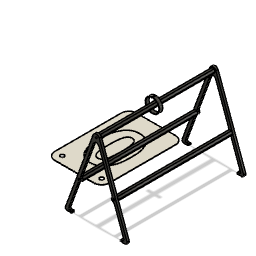
230527 flip scoreboard (Autodesk Fusion 360 design; units mm, degrees)
Autodesk Fusion 360 part; units mm, degrees
sketch "number base" plane through (0, 0, 0) normal (0, 1, 0) x (1, 0, 0)
  line L0 (-14, 0) -> (-86, 0)
  line L1 (-100, -14) -> (-100, -136)
  line L2 (-86, -150) -> (-14, -150)
  line L3 (0, -136) -> (0, -14)
  arc A0 (-14, -150) -> (0, -136) centre (-14, -136) ccw
  arc A1 (-100, -136) -> (-86, -150) centre (-86, -136) ccw
  arc A2 (-86, 0) -> (-100, -14) centre (-86, -14) ccw
  arc A3 (0, -14) -> (-14, 0) centre (-14, -14) ccw
  circle A4 centre (-14, -136) radius 3.5
  circle A5 centre (-86, -136) radius 3.5
  point P0 (-100, 0)
  point P1 (0, -150)
  dimension "d1" = 150
  dimension "d2" = 100
  dimension "d3" = 14
  dimension "d4" = 7
  dimension "d5" = 7
  constraint horizontal L0
  constraint vertical L1
  constraint horizontal L2
  constraint vertical L3
  constraint coincident P1 L2
  constraint coincident P1 L3
  constraint tangent L2 A0
  constraint tangent L3 A0
  constraint tangent L1 A1
  constraint tangent L2 A1
  constraint equal A0 A1
  constraint coincident P0 L0
  constraint coincident P0 L1
  constraint tangent L0 A2
  constraint tangent L1 A2
  constraint equal A0 A2
  constraint coincident origin L0
  constraint coincident origin L3
  constraint tangent L0 A3
  constraint tangent L3 A3
  constraint equal A0 A3
  constraint concentric A0 A4
  constraint concentric A1 A5
  measures "d1" distance of origin P1
  measures "d2" distance of origin P0
  measures "d3" radius of A0
  measures "d4" diameter of A4
  measures "d5" diameter of A5
extrude "Extrude1" add sketch "number base" along normal blind 0.6 makes body 1
sketch "Sketch3" plane through (0, 0.6, 0) normal (0, 1, 0) x (-1, 0, 0)
  circle A0 centre (14, 136) radius 3.5
  circle A1 centre (86, 136) radius 3.5
  arc A2 (0, 14) -> (14, 0) centre (14, 14) ccw
  line L0 (14, 0) -> (86, 0)
  arc A3 (86, 0) -> (100, 14) centre (86, 14) ccw
  line L1 (100, 14) -> (100, 136)
  arc A4 (100, 136) -> (86, 150) centre (86, 136) ccw
  line L2 (86, 150) -> (14, 150)
  arc A5 (14, 150) -> (0, 136) centre (14, 136) ccw
  line L3 (0, 136) -> (0, 14)
  line L4 (0, 75) -> (100, 75)
  line L5 (50, 150) -> (50, 0)
  line L6 (21.099, 26.201) -> (78.901, 26.201) construction
  line L7 (78.901, 26.201) -> (78.901, 123.799) construction
  line L8 (78.901, 123.799) -> (21.099, 123.799) construction
  line L9 (21.099, 123.799) -> (21.099, 26.201) construction
  dimension "d9" = 90
  text T0 "0" font "Arial" height 90 bold align centre middle in box 57.802 x 97.5981 at (21.099, 26.201) x (1, 0) y (0, 1) spacing 1 kerned
  constraint midpoint L3 L4.start
  constraint midpoint L1 L4.end
  constraint midpoint L2 L5.start
  constraint midpoint L0 L5.end
extrude "Extrude2" add sketch "Sketch3" along normal blind 0.4 separate body text T0 makes body 2
combine "Combine1" operation add target body 2 tool bodies 1
sketch "stand" plane through (0, 0, 0) normal (0, 0, 1) x (1, 0, 0)
  line L0 (1.7096, 4.6971) -> (52.5053, 144.257)
  line L1 (4.9985, 0) -> (170, 0) construction
  line L2 (58.1434, 159.7477) -> (58.1434, -80)
  line L3 (4.9985, 0) -> (13, 0)
  line L4 (14, 1) -> (14, 2)
  line L5 (13, 3) -> (9.2691, 3)
  arc A0 (1.7096, 4.6971) -> (4.9985, 0) centre (4.9985, 3.5) ccw
  arc A1 (7.3897, 5.684) -> (9.2691, 3) centre (9.2691, 5) ccw
  arc A2 (14, 2) -> (13, 3) centre (13, 2) ccw
  arc A3 (13, 0) -> (14, 1) centre (13, 1) ccw
  line L6 (103.2868, 3) -> (107.0178, 3)
  arc A4 (103.2868, 3) -> (102.2868, 2) centre (103.2868, 2) ccw
  line L7 (102.2868, 1) -> (102.2868, 2)
  arc A5 (102.2868, 1) -> (103.2868, 0) centre (103.2868, 1) ccw
  line L8 (111.2883, 0) -> (103.2868, 0)
  arc A6 (111.2883, 0) -> (114.5773, 4.6971) centre (111.2883, 3.5) ccw
  line L9 (114.5773, 4.6971) -> (63.7816, 144.257)
  line L10 (108.8971, 5.684) -> (63.3117, 130.9289)
  arc A7 (107.0178, 3) -> (108.8971, 5.684) centre (107.0178, 5) ccw
  arc A8 (63.7816, 144.257) -> (52.5053, 144.257) centre (58.1434, 142.2049) ccw
  arc A9 (63.3117, 130.9289) -> (52.9751, 130.9289) centre (58.1434, 129.0478) ccw
  circle A10 centre (58.1434, 142.2049) radius 1.65
  circle A11 centre (26.0949, 60) radius 1.65
  line L11 (29.1691, 68.4463) -> (23.0207, 51.5537) construction
  line L12 (7.3897, 5.684) -> (24.8987, 53.7896)
  line L13 (29.1705, 65.5264) -> (52.9751, 130.9289)
  arc A12 (27.3762, 56.2108) -> (29.5121, 62.0791) centre (26.0949, 60) ccw
  line L14 (29.8537, 58.6319) -> (32.665, 66.3559) construction
  arc A13 (29.1705, 65.5264) -> (29.5121, 62.0791) centre (32.9293, 64.1583) ccw
  arc A14 (27.3762, 56.2108) -> (24.8987, 53.7896) centre (28.6575, 52.4215) ccw
  point P0 (14, 0)
  dimension "d12" = 70
  dimension "d13" = 170
  dimension "d14" = 14
  dimension "d15" = 5
  dimension "d16" = 3
  dimension "d18" = 3.5
  dimension "d19" = 2
  dimension "d20" = 1
  dimension "d21" = 6
  dimension "d22" = 5.5
  dimension "d23" = 3.3
  dimension "d24" = 3.3
  dimension "d26" = 4
  dimension "d27" = 4
  dimension "d28" = 4
  dimension "d29" = 60
  constraint horizontal L1
  constraint vertical L2
  constraint parallel L1 L3
  constraint perpendicular L1 L4
  constraint perpendicular L4 L5
  constraint parallel L0 L12
  constraint coincident origin L0
  constraint coincident origin L1
  constraint tangent L0 A0
  constraint tangent L1 A0
  constraint tangent L5 A1
  constraint tangent A1 L12
  constraint tangent L4 A2
  constraint tangent L5 A2
  constraint coincident P0 L3
  constraint coincident P0 L4
  constraint tangent L3 A3
  constraint tangent L4 A3
  constraint equal A2 A3
  constraint symmetric L2 L0.start A6.end
  constraint symmetric L2 L1.start L8.start
  constraint symmetric L2 A0 A6
  constraint symmetric L2 L5.end L6.end
  constraint symmetric L2 A1.start L10.start
  constraint symmetric L2 A1 A7
  constraint symmetric L2 L4.end A4.end
  constraint symmetric L2 L5.start L6.start
  constraint symmetric L2 A2 A4
  constraint symmetric L2 L3.end A5.end
  constraint symmetric L2 L4.start L7.start
  constraint symmetric L2 A3 A5
  constraint coincident L2.start L0
  constraint tangent L0 A8
  constraint tangent L9 A8
  constraint tangent A9 L12
  constraint tangent L10 A9
  constraint concentric A8 A10
  constraint symmetric L0 L2 L9
  constraint parallel L0 L11
  constraint collinear L12 L13
  constraint coincident A11.centre L11
  constraint midpoint A11.centre L11
  constraint tangent A12 L14
  constraint parallel L0 L14
  constraint coincident A11.centre A12.centre
  constraint coincident A12 L14.start
  constraint tangent L13 A13
  constraint tangent A12 A13
  constraint tangent L12 A14
  constraint tangent A12 A14
  measures "d12" angle of L0 L1
  measures "d13" distance of origin L2.start
  measures "d14" distance of origin P0
  measures "d15" distance of L0 L12
  measures "d16" distance of L1 L5
  measures "d18" radius of A0
  measures "d19" radius of A1
  measures "d20" radius of A2
  measures "d21" radius of A8
  measures "d22" radius of A9
  measures "d23" diameter of A10
  measures "d24" diameter of A11
  measures "d26" radius of A12
  measures "d27" radius of A13
  measures "d28" radius of A14
  measures "d29" distance of L1 A11.centre
extrude "Extrude3" add sketch "stand" along normal blind 4 separate body contours L0 L2 L3 L4 L5 A0 A1 A2 A3 A8 A9 A10 L12 L13 A12 A13 A14 makes body 3
ref_plane "WorkPlane1" through (58.1434, 137.5514, 2) normal (1, 0, 0) x (0, 1, 0)
mirror "Mirror1" about plane through (58.1434, 137.5514, 2) normal (1, 0, 0) of bodies 3 merged
sketch "shaft" plane through (0, 0, 4) normal (0, 0, 1) x (1, 0, 0)
  arc A0 (63.7816, 144.257) -> (52.5053, 144.257) centre (58.1434, 142.2049) ccw
  line L0 (52.5053, 144.257) -> (1.7096, 4.6971)
  arc A1 (1.7096, 4.6971) -> (4.9985, 0) centre (4.9985, 3.5) ccw
  line L1 (4.9985, 0) -> (13, 0)
  arc A2 (13, 0) -> (14, 1) centre (13, 1) ccw
  line L2 (14, 1) -> (14, 2)
  arc A3 (14, 2) -> (13, 3) centre (13, 2) ccw
  line L3 (13, 3) -> (9.2691, 3)
  arc A4 (7.3897, 5.684) -> (9.2691, 3) centre (9.2691, 5) ccw
  line L4 (7.3897, 5.684) -> (24.8987, 53.7896)
  arc A5 (27.3762, 56.2108) -> (24.8987, 53.7896) centre (28.6575, 52.4215) ccw
  arc A6 (27.3762, 56.2108) -> (29.5121, 62.0791) centre (26.0949, 60) ccw
  arc A7 (29.1705, 65.5264) -> (29.5121, 62.0791) centre (32.9293, 64.1583) ccw
  line L5 (29.1705, 65.5264) -> (52.9751, 130.9289)
  arc A8 (63.3117, 130.9289) -> (52.9751, 130.9289) centre (58.1434, 129.0478) ccw
  line L6 (63.3117, 130.9289) -> (87.1163, 65.5264)
  arc A9 (86.7747, 62.0791) -> (87.1163, 65.5264) centre (83.3575, 64.1583) ccw
  arc A10 (86.7747, 62.0791) -> (88.9106, 56.2108) centre (90.1919, 60) ccw
  arc A11 (91.3881, 53.7896) -> (88.9106, 56.2108) centre (87.6294, 52.4215) ccw
  line L7 (91.3881, 53.7896) -> (108.8971, 5.684)
  arc A12 (107.0178, 3) -> (108.8971, 5.684) centre (107.0178, 5) ccw
  line L8 (107.0178, 3) -> (103.2868, 3)
  arc A13 (103.2868, 3) -> (102.2868, 2) centre (103.2868, 2) ccw
  line L9 (102.2868, 2) -> (102.2868, 1)
  arc A14 (102.2868, 1) -> (103.2868, 0) centre (103.2868, 1) ccw
  line L10 (103.2868, 0) -> (111.2883, 0)
  arc A15 (111.2883, 0) -> (114.5773, 4.6971) centre (111.2883, 3.5) ccw
  line L11 (114.5773, 4.6971) -> (63.7816, 144.257)
  circle A16 centre (90.1919, 60) radius 1.65
  circle A17 centre (26.0949, 60) radius 1.65
  circle A18 centre (58.1434, 142.2049) radius 1.65
  circle A19 centre (58.1434, 142.2049) radius 1.65
  circle A20 centre (58.1434, 142.2049) radius 2.1
  line L12 (60.2434, 145.8422) -> (56.0434, 145.8422)
  line L13 (56.0434, 145.8422) -> (53.9434, 142.2049)
  line L14 (53.9434, 142.2049) -> (56.0434, 138.5676)
  line L15 (56.0434, 138.5676) -> (60.2434, 138.5676)
  line L16 (60.2434, 138.5676) -> (62.3434, 142.2049)
  line L17 (62.3434, 142.2049) -> (60.2434, 145.8422)
  line L18 (58.1434, 142.2049) -> (84, 142.2049) construction
  point P0 (58.1434, 142.2049)
  dimension "d35" = 4.2
  dimension "d36" = 4.2
  constraint concentric A0 A20
  constraint coincident P0 A0.centre
  constraint horizontal L18
  constraint parallel L12 L18
  measures "d35" diameter of A20
  measures "d36" distance of L12.start P0
extrude "Extrude4" add sketch "shaft" along normal blind 210 separate body contours A18 A19 | A20 | L12 L13 L14 L15 L16 L17 makes body 4
extrude "Extrude5" cut sketch "shaft" along normal blind 4.5 contours A18 A19 | A20 bodies 4
ref_plane "WorkPlane2" through (58.1434, 142.2049, 109) normal (0, 0, 1) x (1, 0, 0)
mirror "Mirror2" about plane through (58.1434, 142.2049, 109) normal (0, 0, 1) of "Extrude5"
mirror "Mirror3" about plane through (58.1434, 142.2049, 109) normal (0, 0, 1) of bodies 3 makes body 5
copy_body "CopyPasteBodies2" bodies 4 makes body 6
move_body "Move2" bodies 6 to x (1, 0, 0) y (0, 1, 0) z (0, 0, 1) at (-31.8011, -82.3439, 0)
copy_body "CopyPasteBodies3" bodies 6 makes body 7
move_body "Move3" bodies 7 to x (1, 0, 0) y (0, 1, 0) z (0, 0, 1) at (64, 0, 0)
sketch "Sketch6" plane through (58.1434, 142.2049, 109) normal (0, 0, 1) x (1, 0, 0)
  line L0 (0, 0) -> (0, 13) construction
  line L1 (0, 0) -> (-0.1815, 12.9987) construction
  line L2 (0, 12) -> (0, 13)
  line L3 (-0.1675, 11.9988) -> (-0.1815, 12.9987)
  arc A0 (-0.1815, 12.9987) -> (0.6, 12.9861) centre (0, 0) ccw
  arc A1 (-0.1675, 11.9988) -> (0, 12) centre (0, 0) ccw
  line L4 (0.6, 12.9861) -> (0.6, 13.7)
  line L5 (0.6, 13.7) -> (0, 13.7)
  line L6 (0, 13.7) -> (0, 13)
  dimension "d45" = 26
  dimension "d46" = 24
  dimension "d47" = 0.8
  dimension "d71" = 0.7
  dimension "d76" = 0.6
  constraint coincident L0.start L1.start
  constraint concentric A0 A1
  constraint vertical L0
  constraint coincident L0 L2.start
  constraint parallel L0 L2
  constraint coincident L1 L3.start
  constraint vertical L4
  constraint horizontal L5
  constraint vertical L6
  measures "d45" diameter of A0
  measures "d46" diameter of A1
  measures "d47" angle of L0 L1
  measures "d71" distance of L0.end L5.end
  measures "d76" distance of L4.end L5.end
extrude "Extrude6" add sketch "Sketch6" along normal blind 6 separate body makes body 8
fillet "Fillet8" radius 0.2 2 edges at (58.7434, 155.9049, 112) (58.7434, 155.1911, 112) on bodies 8
fillet "Fillet9" radius 0.2 1 edges at (58.1434, 155.9049, 112) on bodies 8
fillet "Fillet7" [suppressed]
fillet "Fillet6" [suppressed]
named bodies: "number base", "number plate", "stand left", "shaft", "stand right", "shaft lower 2", "shaft (1)", "shaft lower 1", "ring"
